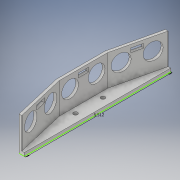
# Autodesk Inventor part: UltrasonicSensorMountSingle
Saved by Autodesk Inventor 2019 (Build 230136000, 136)
## iProperties
Created: 2020-06-23
Part Number: UltrasonicSensorMountSingle
Material: Generic
Document SubType Name: Modeling
Designer: garretthagen21
Density: 1 g/cm^3
Appearance: Default
Author: garretthagen21
Autodesk Inventor part; units mm, degrees
ref_plane "YZ Plane" through (0, 0, 0) normal (1, 0, 0) x (0, 1, 0)
ref_plane "XZ Plane" through (0, 0, 0) normal (0, 1, 0) x (-1, 0, 0)
ref_plane "XY Plane" through (0, 0, 0) normal (0, 0, 1) x (1, 0, 0)
sketch "Base" plane through (0, 0, 0) normal (0, 1, 0) x (-1, 0, 0)
  line L0 (-10.6945, 15.9529) -> (-10.6945, -124.0471)
  line L1 (5.3055, -77.3796) -> (5.3055, -30.7069)
  line L2 (-10.6945, 15.9529) -> (-5.6266, 15.9529)
  line L3 (-5.6266, 15.9529) -> (5.3055, -30.7069)
  line L4 (-10.6945, -124.0471) -> (-5.6266, -124.0471)
  line L5 (5.3055, -77.3796) -> (-5.6266, -124.0471)
  point P0 (0, 0)
  dimension "d1" = 140
  constraints: 12 end point, 1 parallel
  measures "d1" distance of L0.end L0.start
extrude "Extrusion1" add sketch "Base" along normal blind 3
sketch "FrontWall" plane through (0, 3, 0) normal (0, 1, 0) x (1, 0, 0)
  line L0 (-5.3055, 30.7069) -> (5.6266, -15.9529) projected
  line L1 (-5.3055, 77.3796) -> (-5.3055, 30.7069) projected
  line L2 (5.6266, 124.0471) -> (-5.3055, 77.3796) projected
  line L3 (8.0997, -15.3735) -> (-2.7655, 31.0004)
  line L4 (-2.7655, 31.0004) -> (-2.7655, 77.0861)
  line L5 (-2.7655, 77.0861) -> (8.0997, 123.4677)
  line L6 (8.0997, -15.3735) -> (8.1606, -15.9529)
  line L7 (5.6266, -15.9529) -> (10.6945, -15.9529) projected
  line L8 (8.0997, 123.4677) -> (8.0997, 124.0471)
  line L9 (10.6945, 124.0471) -> (5.6266, 124.0471) projected
  point P0 (0, 0)
  dimension "d6" = 2.54
  constraints: 10 end point, 1 midpoint, 1 point on line, 1 vertical, 2 other
  measures "d6" distance between parallel lines of L0 L3
extrude "Extrusion2" add sketch "FrontWall" along normal blind 29.464
sketch "Sketch3" plane through (-5.3055, 0, -77.3796) normal (-0.9736421, 0, -0.2280812) x (-0.2280812, 0, 0.9736421)
  line L0 (-47.9308, 0) -> (-47.9308, 32.464) projected
  line L1 (0, 0) -> (0, 32.464) projected
  line L2 (-1.0536, 30.5772) -> (-46.5036, 30.5772)
  line L3 (-46.5036, 30.5772) -> (-46.5036, 10.0772)
  line L4 (-46.5036, 10.0772) -> (-1.0536, 10.0772)
  line L5 (-1.0536, 10.0772) -> (-1.0536, 30.5772)
  line L6 (-23.7786, 29.5772) -> (-28.8286, 29.5772)
  line L7 (-28.8286, 29.5772) -> (-28.8286, 25.6172)
  line L8 (-28.8286, 25.6172) -> (-18.7194, 25.6172)
  line L9 (-18.7194, 25.6172) -> (-18.7194, 29.5772)
  line L10 (-18.7194, 29.5772) -> (-23.7786, 29.5772)
  point P0 (74.13, 0)
  point P1 (-36.5036, 20.3272)
  point P2 (-11.0612, 20.3272)
  dimension "d9" = 47.9308
  dimension "d10" = 45.45
  dimension "d11" = 20.5
  constraints: 18 end point, 5 perpendicular, 3 parallel, 1 horizontal, 1 point on line
  measures "d9" distance between parallel lines of L0 L1
  measures "d10" distance of L4.end L3.end
  measures "d11" distance of L2.end L3.end
hole "Hole1" at (-2.7826, 20.3272, -88.1493) at (3.0203, 20.3272, -112.9211) direction (0.9736421, 0, 0.2280812) diameter 16 end through all
extrude "Extrusion3" cut sketch "Sketch3" against normal blind 29.464 contours L10 L9 L8 L7 L6
sketch "Sketch4" plane through (-5.3055, 0, -77.3796) normal (-1, 0, 0) x (0, 0, 1)
  point P0 (77.3796, 0)
sketch "Sketch5" plane through (-5.3055, 0, -77.3796) normal (-1, 0, 0) x (0, 0, 1)
  line L0 (-47.9308, 0) -> (-47.9308, 32.464)
  line L1 (0, 0) -> (0, 32.464)
  line L2 (46.1641, 30.5772) -> (0.7141, 30.5772)
  line L3 (0.7141, 30.5772) -> (0.7141, 10.0772)
  line L4 (0.7141, 10.0772) -> (46.1641, 10.0772)
  line L5 (46.1641, 10.0772) -> (46.1641, 30.5772)
  line L6 (23.4391, 29.5772) -> (18.3891, 29.5772)
  line L7 (18.3891, 29.5772) -> (18.3891, 25.6172)
  line L8 (18.3891, 25.6172) -> (28.4983, 25.6172)
  line L9 (28.4983, 25.6172) -> (28.4983, 29.5772)
  line L10 (28.4983, 29.5772) -> (23.4391, 29.5772)
  point P0 (77.3796, 0)
  point P1 (74.13, 0)
  point P2 (10.7141, 20.3272)
  point P3 (36.1565, 20.3272)
  dimension "d27" = 47.9308
  dimension "d28" = 45.45
  dimension "d29" = 20.5
  constraints: 22 end point, 5 perpendicular, 3 parallel, 1 horizontal, 1 point on line
  measures "d27" distance between parallel lines of L0 L1
  measures "d28" distance of L4.end L3.end
  measures "d29" distance of L2.end L3.end
hole "Hole2" at (-5.3055, 20.3272, -41.2231) at (-5.3055, 20.3272, -66.6655) direction (1, 0, 0) diameter 16 end through all
extrude "Extrusion4" cut sketch "Sketch5" against normal blind 29.464 contours L10 L9 L8 L7 L6
sketch "Sketch6" plane through (5.6266, 0, 15.9529) normal (-0.9736338, 0, 0.2281165) x (0.2281165, 0, 0.9736338)
  line L0 (-47.9308, 0) -> (-47.9308, 32.464)
  line L1 (-47.1544, 0) -> (-47.1544, 32.464)
  line L2 (-0.9903, 30.5772) -> (-46.4403, 30.5772)
  line L3 (-46.4403, 30.5772) -> (-46.4403, 10.0772)
  line L4 (-46.4403, 10.0772) -> (-0.9903, 10.0772)
  line L5 (-0.9903, 10.0772) -> (-0.9903, 30.5772)
  line L6 (-23.7153, 29.5772) -> (-28.7653, 29.5772)
  line L7 (-28.7653, 29.5772) -> (-28.7653, 25.6172)
  line L8 (-28.7653, 25.6172) -> (-18.6561, 25.6172)
  line L9 (-18.6561, 25.6172) -> (-18.6561, 29.5772)
  line L10 (-18.6561, 29.5772) -> (-23.7153, 29.5772)
  point P0 (-16.8159, 0)
  point P1 (77.3796, 0)
  point P2 (74.13, 0)
  point P3 (-36.4403, 20.3272)
  point P4 (-10.9979, 20.3272)
  dimension "d39" = 0.7874
  dimension "d40" = 45.45
  dimension "d41" = 20.5
  constraints: 22 end point, 5 perpendicular, 3 parallel, 1 horizontal, 1 point on line
  measures "d40" distance of L4.end L3.end
  measures "d41" distance of L2.end L3.end
hole "Hole3" at (-2.686, 20.3272, -19.5266) at (3.1178, 20.3272, 5.245) direction (0.9736338, 0, -0.2281165) diameter 16 end through all
extrude "Extrusion5" cut sketch "Sketch6" against normal blind 29.464 contours L10 L9 L8 L7 L6
sketch "Sketch7" plane through (0, 3, 0) normal (0, 1, 0) x (1, 0, 0)
  line L0 (10.6945, 124.0471) -> (10.6945, -15.9529) projected
  point P0 (0, 0)
  point P1 (2.8129, 67.1471)
  point P2 (2.8129, 40.9471)
hole "Hole4" at (2.8129, 3, -40.9471) at (2.8129, 3, -67.1471) direction (0, -1, 0) diameter 4 end through all
body "Solid1"
